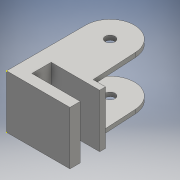
# Autodesk Inventor part: Maintients poullie v1
Saved by Autodesk Inventor 2016 (Build 200138000, 138)
## iProperties
Created: 2016-02-22
Part Number: Maintients poullie v1
Material: Generic
Document SubType Name: Modeling
Designer: Thetheos
Density: 1 g/cm^3
Appearance: Default
Author: Thetheos
Autodesk Inventor part; units mm, degrees
ref_plane "YZ Plane" through (0, 0, 0) normal (1, 0, 0) x (0, 1, 0)
ref_plane "XZ Plane" through (0, 0, 0) normal (0, 1, 0) x (-1, 0, 0)
ref_plane "XY Plane" through (0, 0, 0) normal (0, 0, 1) x (1, 0, 0)
sketch "Sketch1" plane through (0, 0, 0) normal (0, 0, 1) x (1, 0, 0)
  line L0 (0, 0) -> (26.1364, 0)
  line L1 (26.1364, 0) -> (26.1364, 4.2728)
  line L2 (26.1364, 4.2728) -> (6.1364, 4.2728)
  line L3 (6.1364, 4.2728) -> (6.1364, 12.2728)
  line L4 (6.1364, 12.2728) -> (26.1364, 12.2728)
  line L5 (26.1364, 12.2728) -> (26.1364, 14.7274)
  line L6 (26.1364, 14.7274) -> (0, 14.7274)
  line L7 (0, 14.7274) -> (0, 0)
  line L8 (0, 14.7274) -> (0, 32.7274)
  arc A0 (19.9894, 33.187) -> (0, 32.7274) centre (10, 32.7274) ccw
  line L9 (19.9894, 33.187) -> (21, 14.7274)
  circle A1 centre (10, 32.7274) radius 2
  dimension "d0" = 20
  dimension "d1" = 8
  dimension "d3" = 4
  dimension "d4" = 10
  dimension "d5" = 18
  dimension "d7" = 19.9894
  constraints: 20 end point, 6 perpendicular, 3 point on line, 2 centre point, 2 point on circle, 1 coincident, 1 tangent
  measures "d0" distance of L3.end L4.end
  measures "d1" distance of L2.end L3.end
  measures "d3" diameter of A1
  measures "d4" distance from line of A0.centre L8
  measures "d5" distance from line of L6 A0.centre
  measures "d7" horizontal distance of L9.start L8.end
extrude "Extrusion1" add sketch "Sketch1" along normal blind 22
sketch "Sketch2" plane through (19.9894, 33.187, 22) normal (0.9985049, 0.0546629, 0) x (0, 0, -1)
  line L0 (1.8448, -6.1786) -> (1.8448, -17.437)
  line L1 (20.3448, -6.1786) -> (20.3448, -17.437)
  line L2 (20.3448, -17.437) -> (1.8448, -17.437)
  line L3 (1.8448, -6.1786) -> (1.8448, 10.563)
  line L4 (1.8448, 10.563) -> (20.3448, 10.563)
  line L5 (20.3448, 10.563) -> (20.3448, -6.1786)
  dimension "d14" = 28
  dimension "d17" = 18.5
  constraints: 12 end point, 2 perpendicular, 1 collinear, 1 point on line
  measures "d14" distance between parallel lines of L2 L4
  measures "d17" distance between parallel lines of L5 L3
extrude "Extrusion2" cut sketch "Sketch2" against normal through all
sketch "Sketch3" plane through (19.9894, 33.187, 22) normal (-0.9985049, -0.0546629, 0) x (0, 0, 1)
  line L0 (-20.3448, 0.1742) -> (-1.8448, 0.1742) projected
  line L1 (-1.8448, 0.1742) -> (-17.8448, 0.1742)
  line L2 (-17.8448, 0.1742) -> (-17.8448, -0.1891)
  line L3 (-17.8448, -0.1891) -> (-1.8448, -0.1891)
  line L4 (-1.8448, -0.1891) -> (-1.8448, 0.1742)
  point P0 (-22, -32.0447)
  constraints: 8 end point, 2 parallel, 1 horizontal, 1 perpendicular
extrude "Extrusion3" cut sketch "Sketch3" against normal through all
sketch "Sketch4" plane through (21, 14.7274, 22) normal (0.9985049, 0.0546629, 0) x (0, 0, -1)
  point P0 (22, -13.5574)
sketch "Sketch5" plane through (0, 0, 22) normal (0, 0, 1) x (1, 0, 0)
  point P0 (0, 0)
sketch "Sketch6" plane through (0, 0, 0) normal (0, 0, -1) x (-1, 0, 0)
  point P0 (0, 0)
sketch "Sketch7" plane through (0, 0, 22) normal (0, 0, 1) x (1, 0, 0)
  point P0 (0, 0)
sketch "Sketch8" plane through (19.9894, 33.187, 22) normal (-0.9985049, -0.0546629, 0) x (0, 0, 1)
  point P0 (-22, -32.0447)
sketch "Sketch9" plane through (19.9894, 33.187, 22) normal (-0.9985049, -0.0546629, 0) x (0, 0, 1)
  line L0 (-20.3448, 0) -> (-20.3448, -17.437) projected
  line L1 (-20.3448, 0.1742) -> (-17.8448, 0.1742) projected
  line L2 (-20.3448, 0) -> (-17.8448, 0)
  line L3 (-17.8448, 0) -> (-17.8448, 0.1742)
  line L4 (-17.8448, 0.1742) -> (-20.3448, 0.1742)
  line L5 (-20.3448, 0.1742) -> (-20.3448, 0)
  point P0 (-22, -32.0447)
  constraints: 8 end point, 2 parallel, 1 horizontal, 1 perpendicular
extrude "Extrusion4" cut sketch "Sketch9" against normal through all
body "Solid1"
